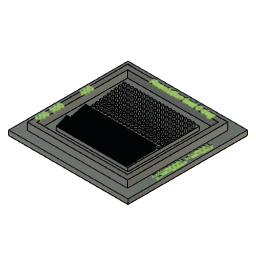
resolution_test_plate_increasing_feature_size v6 (Autodesk Fusion 360 design; units mm, degrees)
Autodesk Fusion 360 part; units mm, degrees
note: some values were not read from the file. Set by a fixed rule: which face or edge a step refers to.
(part 1 of 2)
sketch "Sketch1" plane through (0, 0, 0) normal (0, 0, 1) x (1, 0, 0)
  line L0 (0, 0) -> (-25, 0)
  line L1 (-25, 0) -> (-25, 25)
  line L2 (-25, 25) -> (0, 25)
  line L3 (0, 25) -> (0, 0)
  dimension "d1" = 25
  dimension "d2" = 25
  constraint horizontal L0
  constraint vertical L1
  constraint horizontal L2
  constraint vertical L3
  constraint coincident L0.start L3.end
  measures "d1" distance of L0.start L0.end
  measures "d2" distance of L0.start L2.end
extrude "Extrude1" add sketch "Sketch1" along normal blind 1
sketch "Sketch2" plane through (0, 0, 1) normal (0, 0, 1) x (-1, 0, 0)
  line L0 (0, -25) -> (25, -25)
  line L1 (25, -25) -> (25, 0)
  line L2 (25, 0) -> (0, 0)
  line L3 (0, 0) -> (0, -25)
  line L4 (22.9884, -22.8968) -> (1.9884, -22.8968)
  line L5 (1.9884, -22.8968) -> (1.9884, -1.8968)
  line L6 (1.9884, -1.8968) -> (22.9884, -1.8968)
  line L7 (22.9884, -1.8968) -> (22.9884, -22.8968)
  dimension "d5" = 21
  dimension "d6" = 21
  constraint horizontal L4
  constraint vertical L5
  constraint horizontal L6
  constraint vertical L7
  measures "d5" distance of L4.start L4.end
  measures "d6" distance of L4.start L6.end
extrude "Extrude2" add sketch "Sketch2" along normal blind 1.5 contours L4 L5 L6 L7
shell "Shell1" thickness 1 removed faces 1 at (-15.9884, 15.8968, 2.5)
sketch "Sketch3" plane through (0, 0, 1) normal (0, 0, 1) x (-1, 0, 0)
  line L0 (21.9884, -2.8968) -> (2.9884, -2.8968)
  line L1 (2.9884, -2.8968) -> (2.9884, -21.8968)
  line L2 (2.9884, -21.8968) -> (21.9884, -21.8968)
  line L3 (21.9884, -21.8968) -> (21.9884, -2.8968)
  line L4 (19.953, -19.9105) -> (4.953, -19.9105)
  line L5 (4.953, -19.9105) -> (4.953, -4.9105)
  line L6 (4.953, -4.9105) -> (19.953, -4.9105)
  line L7 (19.953, -4.9105) -> (19.953, -19.9105)
  dimension "d10" = 15
  dimension "d11" = 15
  constraint horizontal L4
  constraint vertical L5
  constraint horizontal L6
  constraint vertical L7
  measures "d10" distance of L4.start L4.end
  measures "d11" distance of L4.start L6.end
extrude "Extrude3" add sketch "Sketch3" along normal blind 0.75 contours L4 L5 L6 L7
sketch "Sketch6" plane through (0, 0, 1.75) normal (0, 0, 1) x (-1, 0, 0)
  line L0 (19.953, -4.9105) -> (4.953, -4.9105)
  line L1 (4.953, -4.9105) -> (4.953, -19.9105)
  line L2 (4.953, -19.9105) -> (19.953, -19.9105)
  line L3 (19.953, -19.9105) -> (19.953, -4.9105)
  line L4 (19.8995, -4.9499) -> (19.7995, -4.9499)
  line L5 (19.7995, -4.9499) -> (19.7995, -5.0499)
  line L6 (19.7995, -5.0499) -> (19.8995, -5.0499)
  line L7 (19.8995, -5.0499) -> (19.8995, -4.9499)
  dimension "d88" = 0.1
  dimension "d89" = 0.1
  constraint horizontal L4
  constraint vertical L5
  constraint horizontal L6
  constraint vertical L7
  measures "d88" distance of L4.start L4.end
  measures "d89" distance of L4.start L6.end
extrude "Extrude10" add sketch "Sketch6" along normal blind 0.1 contours L4 L5 L6 L7
pattern_linear "R-Pattern10" count 10 spacing 0.2222 along (0, 1, 0) of 5 faces at (-19.8662, 4.9499, 1.7833) (-19.8328, 5.0165, 1.85) (-19.7995, 4.9832, 1.7833) (-19.8328, 5.0499, 1.7833) (-19.8995, 5.0165, 1.7833)
extrude "Extrude11" add 1 faces at (-19.8328, 5.2387, 1.85) along direction (0, 0, 1) blind 0.1
extrude "Extrude12" add 1 faces at (-19.8328, 5.461, 1.85) along direction (0, 0, 1) blind 0.2
extrude "Extrude13" add 1 faces at (-19.8328, 5.6832, 1.85) along direction (0, 0, 1) blind 0.3
extrude "Extrude14" add 1 faces at (-19.8328, 5.9054, 1.85) along direction (0, 0, 1) blind 0.4
extrude "Extrude15" add 1 faces at (-19.8328, 6.1276, 1.85) along direction (0, 0, 1) blind 0.5
extrude "Extrude16" add 1 faces at (-19.8328, 6.3499, 1.85) along direction (0, 0, 1) blind 0.6
extrude "Extrude17" add 1 faces at (-19.8328, 6.5721, 1.85) along direction (0, 0, 1) blind 0.7
extrude "Extrude18" add 1 faces at (-19.8328, 6.7943, 1.85) along direction (0, 0, 1) blind 0.8
extrude "Extrude19" add 1 faces at (-19.8328, 7.0165, 1.85) along direction (0, 0, 1) blind 0.9
sketch "Sketch7" plane through (0, 0, 1.75) normal (0, 0, 1) x (-1, 0, 0)
  line L0 (19.8995, -7.0499) -> (19.7995, -7.0499)
  line L1 (19.7995, -7.0499) -> (19.7995, -6.9499)
  line L2 (19.7995, -6.9499) -> (19.8995, -6.9499)
  line L3 (19.8995, -6.9499) -> (19.8995, -7.0499)
  line L4 (19.8995, -6.8276) -> (19.7995, -6.8276)
  line L5 (19.7995, -6.8276) -> (19.7995, -6.7276)
  line L6 (19.7995, -6.7276) -> (19.8995, -6.7276)
  line L7 (19.8995, -6.7276) -> (19.8995, -6.8276)
  line L8 (19.8995, -6.6054) -> (19.7995, -6.6054)
  line L9 (19.7995, -6.6054) -> (19.7995, -6.5054)
  line L10 (19.7995, -6.5054) -> (19.8995, -6.5054)
  line L11 (19.8995, -6.5054) -> (19.8995, -6.6054)
  line L12 (19.8995, -6.3832) -> (19.7995, -6.3832)
  line L13 (19.7995, -6.3832) -> (19.7995, -6.2832)
  line L14 (19.7995, -6.2832) -> (19.8995, -6.2832)
  line L15 (19.8995, -6.2832) -> (19.8995, -6.3832)
  line L16 (19.8995, -6.161) -> (19.7995, -6.161)
  line L17 (19.7995, -6.161) -> (19.7995, -6.061)
  line L18 (19.7995, -6.061) -> (19.8995, -6.061)
  line L19 (19.8995, -6.061) -> (19.8995, -6.161)
  line L20 (19.8995, -5.9387) -> (19.7995, -5.9387)
  line L21 (19.7995, -5.9387) -> (19.7995, -5.8387)
  line L22 (19.7995, -5.8387) -> (19.8995, -5.8387)
  line L23 (19.8995, -5.8387) -> (19.8995, -5.9387)
  line L24 (19.8995, -5.7165) -> (19.7995, -5.7165)
  line L25 (19.7995, -5.7165) -> (19.7995, -5.6165)
  line L26 (19.7995, -5.6165) -> (19.8995, -5.6165)
  line L27 (19.8995, -5.6165) -> (19.8995, -5.7165)
  line L28 (19.8995, -5.4943) -> (19.7995, -5.4943)
  line L29 (19.7995, -5.4943) -> (19.7995, -5.3943)
  line L30 (19.7995, -5.3943) -> (19.8995, -5.3943)
  line L31 (19.8995, -5.3943) -> (19.8995, -5.4943)
  line L32 (19.8995, -5.2721) -> (19.7995, -5.2721)
  line L33 (19.7995, -5.2721) -> (19.7995, -5.1721)
  line L34 (19.7995, -5.1721) -> (19.8995, -5.1721)
  line L35 (19.8995, -5.1721) -> (19.8995, -5.2721)
  line L36 (19.8995, -5.0499) -> (19.7995, -5.0499)
  line L37 (19.7995, -5.0499) -> (19.7995, -4.9499)
  line L38 (19.7995, -4.9499) -> (19.8995, -4.9499)
  line L39 (19.8995, -4.9499) -> (19.8995, -5.0499)
  line L40 (19.953, -4.9105) -> (4.953, -4.9105)
  line L41 (4.953, -4.9105) -> (4.953, -19.9105)
  line L42 (4.953, -19.9105) -> (19.953, -19.9105)
  line L43 (19.953, -19.9105) -> (19.953, -4.9105)
  line L44 (19.8984, -7.2019) -> (19.6984, -7.2019)
  line L45 (19.6984, -7.2019) -> (19.6984, -7.4019)
  line L46 (19.6984, -7.4019) -> (19.8984, -7.4019)
  line L47 (19.8984, -7.4019) -> (19.8984, -7.2019)
  dimension "d122" = 0.2
  dimension "d123" = 0.2
  constraint horizontal L44
  constraint vertical L45
  constraint horizontal L46
  constraint vertical L47
  measures "d122" distance of L44.start L44.end
  measures "d123" distance of L44.start L46.end
extrude "Extrude20" add sketch "Sketch7" along normal blind 0.1 contours L44 L45 L46 L47
pattern_linear "R-Pattern12" count 10 spacing 0.4 along (0, 1, 0) of 5 faces at (-19.8317, 7.2019, 1.7833) (-19.7651, 7.2685, 1.85) (-19.6984, 7.2685, 1.7833) (-19.7651, 7.4019, 1.7833) (-19.8984, 7.3352, 1.7833)
sketch "Sketch8" plane through (0, 0, 1.75) normal (0, 0, 1) x (-1, 0, 0)
  line L0 (19.8984, -11.0019) -> (19.6984, -11.0019)
  line L1 (19.6984, -11.0019) -> (19.6984, -10.8019)
  line L2 (19.6984, -10.8019) -> (19.8984, -10.8019)
  line L3 (19.8984, -10.8019) -> (19.8984, -11.0019)
  line L4 (19.8984, -10.6019) -> (19.6984, -10.6019)
  line L5 (19.6984, -10.6019) -> (19.6984, -10.4019)
  line L6 (19.6984, -10.4019) -> (19.8984, -10.4019)
  line L7 (19.8984, -10.4019) -> (19.8984, -10.6019)
  line L8 (19.8984, -10.2019) -> (19.6984, -10.2019)
  line L9 (19.6984, -10.2019) -> (19.6984, -10.0019)
  line L10 (19.6984, -10.0019) -> (19.8984, -10.0019)
  line L11 (19.8984, -10.0019) -> (19.8984, -10.2019)
  line L12 (19.8984, -9.8019) -> (19.6984, -9.8019)
  line L13 (19.6984, -9.8019) -> (19.6984, -9.6019)
  line L14 (19.6984, -9.6019) -> (19.8984, -9.6019)
  line L15 (19.8984, -9.6019) -> (19.8984, -9.8019)
  line L16 (19.8984, -9.4019) -> (19.6984, -9.4019)
  line L17 (19.6984, -9.4019) -> (19.6984, -9.2019)
  line L18 (19.6984, -9.2019) -> (19.8984, -9.2019)
  line L19 (19.8984, -9.2019) -> (19.8984, -9.4019)
  line L20 (19.8984, -9.0019) -> (19.6984, -9.0019)
  line L21 (19.6984, -9.0019) -> (19.6984, -8.8019)
  line L22 (19.6984, -8.8019) -> (19.8984, -8.8019)
  line L23 (19.8984, -8.8019) -> (19.8984, -9.0019)
  line L24 (19.8984, -8.6019) -> (19.6984, -8.6019)
  line L25 (19.6984, -8.6019) -> (19.6984, -8.4019)
  line L26 (19.6984, -8.4019) -> (19.8984, -8.4019)
  line L27 (19.8984, -8.4019) -> (19.8984, -8.6019)
  line L28 (19.8984, -8.2019) -> (19.6984, -8.2019)
  line L29 (19.6984, -8.2019) -> (19.6984, -8.0019)
  line L30 (19.6984, -8.0019) -> (19.8984, -8.0019)
  line L31 (19.8984, -8.0019) -> (19.8984, -8.2019)
  line L32 (19.8984, -7.8019) -> (19.6984, -7.8019)
  line L33 (19.6984, -7.8019) -> (19.6984, -7.6019)
  line L34 (19.6984, -7.6019) -> (19.8984, -7.6019)
  line L35 (19.8984, -7.6019) -> (19.8984, -7.8019)
  line L36 (19.8984, -7.4019) -> (19.6984, -7.4019)
  line L37 (19.6984, -7.4019) -> (19.6984, -7.2019)
  line L38 (19.6984, -7.2019) -> (19.8984, -7.2019)
  line L39 (19.8984, -7.2019) -> (19.8984, -7.4019)
  line L40 (19.8995, -7.0499) -> (19.7995, -7.0499)
  line L41 (19.7995, -7.0499) -> (19.7995, -6.9499)
  line L42 (19.7995, -6.9499) -> (19.8995, -6.9499)
  line L43 (19.8995, -6.9499) -> (19.8995, -7.0499)
  line L44 (19.8995, -6.8276) -> (19.7995, -6.8276)
  line L45 (19.7995, -6.8276) -> (19.7995, -6.7276)
  line L46 (19.7995, -6.7276) -> (19.8995, -6.7276)
  line L47 (19.8995, -6.7276) -> (19.8995, -6.8276)
  line L48 (19.8995, -6.6054) -> (19.7995, -6.6054)
  line L49 (19.7995, -6.6054) -> (19.7995, -6.5054)
  line L50 (19.7995, -6.5054) -> (19.8995, -6.5054)
  line L51 (19.8995, -6.5054) -> (19.8995, -6.6054)
  line L52 (19.8995, -6.3832) -> (19.7995, -6.3832)
  line L53 (19.7995, -6.3832) -> (19.7995, -6.2832)
  line L54 (19.7995, -6.2832) -> (19.8995, -6.2832)
  line L55 (19.8995, -6.2832) -> (19.8995, -6.3832)
  line L56 (19.8995, -6.161) -> (19.7995, -6.161)
  line L57 (19.7995, -6.161) -> (19.7995, -6.061)
  line L58 (19.7995, -6.061) -> (19.8995, -6.061)
  line L59 (19.8995, -6.061) -> (19.8995, -6.161)
  line L60 (19.8995, -5.9387) -> (19.7995, -5.9387)
  line L61 (19.7995, -5.9387) -> (19.7995, -5.8387)
  line L62 (19.7995, -5.8387) -> (19.8995, -5.8387)
  line L63 (19.8995, -5.8387) -> (19.8995, -5.9387)
  line L64 (19.8995, -5.7165) -> (19.7995, -5.7165)
  line L65 (19.7995, -5.7165) -> (19.7995, -5.6165)
  line L66 (19.7995, -5.6165) -> (19.8995, -5.6165)
  line L67 (19.8995, -5.6165) -> (19.8995, -5.7165)
  line L68 (19.8995, -5.4943) -> (19.7995, -5.4943)
  line L69 (19.7995, -5.4943) -> (19.7995, -5.3943)
  line L70 (19.7995, -5.3943) -> (19.8995, -5.3943)
  line L71 (19.8995, -5.3943) -> (19.8995, -5.4943)
  line L72 (19.8995, -5.2721) -> (19.7995, -5.2721)
  line L73 (19.7995, -5.2721) -> (19.7995, -5.1721)
  line L74 (19.7995, -5.1721) -> (19.8995, -5.1721)
  line L75 (19.8995, -5.1721) -> (19.8995, -5.2721)
  line L76 (19.8995, -5.0499) -> (19.7995, -5.0499)
  line L77 (19.7995, -5.0499) -> (19.7995, -4.9499)
  line L78 (19.7995, -4.9499) -> (19.8995, -4.9499)
  line L79 (19.8995, -4.9499) -> (19.8995, -5.0499)
  line L80 (19.953, -4.9105) -> (4.953, -4.9105)
  line L81 (4.953, -4.9105) -> (4.953, -19.9105)
  line L82 (4.953, -19.9105) -> (19.953, -19.9105)
  line L83 (19.953, -19.9105) -> (19.953, -4.9105)
  line L84 (19.899, -11.503) -> (19.499, -11.503)
  line L85 (19.499, -11.503) -> (19.499, -11.903)
  line L86 (19.499, -11.903) -> (19.899, -11.903)
  line L87 (19.899, -11.903) -> (19.899, -11.503)
  dimension "d130" = 0.4
  dimension "d131" = 0.4
  constraint horizontal L84
  constraint vertical L85
  constraint horizontal L86
  constraint vertical L87
  measures "d130" distance of L84.start L84.end
  measures "d131" distance of L84.start L86.end
extrude "Extrude21" add sketch "Sketch8" along normal blind 0.1 contours L84 L85 L86 L87
pattern_linear "R-Pattern13" count 10 spacing 0.8 along (0, 1, 0) of 5 faces at (-19.6323, 11.6364, 1.85) (-19.7657, 11.503, 1.7833) (-19.499, 11.6364, 1.7833) (-19.6323, 11.903, 1.7833) (-19.899, 11.7697, 1.7833)
extrude "Extrude22" add 1 faces at (-19.7651, 7.6685, 1.85) along direction (0, 0, 1) blind 0.1
extrude "Extrude23" add 1 faces at (-19.7651, 8.0685, 1.85) along direction (0, 0, 1) blind 0.2
extrude "Extrude24" add 1 faces at (-19.7651, 8.4685, 1.85) along direction (0, 0, 1) blind 0.3
extrude "Extrude25" add 1 faces at (-19.7651, 8.8685, 1.85) along direction (0, 0, 1) blind 0.4
extrude "Extrude26" add 1 faces at (-19.7651, 9.2685, 1.85) along direction (0, 0, 1) blind 0.5
extrude "Extrude27" add 1 faces at (-19.7651, 9.6685, 1.85) along direction (0, 0, 1) blind 0.6
extrude "Extrude28" add 1 faces at (-19.7651, 10.0685, 1.85) along direction (0, 0, 1) blind 0.7
extrude "Extrude29" add 1 faces at (-19.7651, 10.4685, 1.85) along direction (0, 0, 1) blind 0.8
extrude "Extrude30" add 1 faces at (-19.7651, 10.8685, 1.85) along direction (0, 0, 1) blind 0.9
extrude "Extrude31" add 1 faces at (-19.6323, 12.4364, 1.85) along direction (0, 0, 1) blind 0.1
extrude "Extrude32" add 1 faces at (-19.6323, 13.2364, 1.85) along direction (0, 0, 1) blind 0.2
extrude "Extrude33" add 1 faces at (-19.6323, 14.0364, 1.85) along direction (0, 0, 1) blind 0.3
extrude "Extrude34" add 1 faces at (-19.6323, 14.8364, 1.85) along direction (0, 0, 1) blind 0.4
extrude "Extrude35" add 1 faces at (-19.6323, 15.6364, 1.85) along direction (0, 0, 1) blind 0.5
extrude "Extrude36" add 1 faces at (-19.6323, 16.4364, 1.85) along direction (0, 0, 1) blind 0.6
extrude "Extrude37" add 1 faces at (-19.6323, 17.2364, 1.85) along direction (0, 0, 1) blind 0.7
extrude "Extrude38" add 1 faces at (-19.6323, 18.0364, 1.85) along direction (0, 0, 1) blind 0.8
extrude "Extrude39" add 1 faces at (-19.6323, 18.8364, 1.85) along direction (0, 0, 1) blind 0.9
pattern_linear "R-Pattern14" count 19 spacing 0.8 along (1, 0, 0) of 50 faces at (-19.6323, 18.703, 2.4167) (-19.499, 18.9697, 2.4167) (-19.6323, 18.8364, 2.75) (-19.499, 18.0364, 2.35) (-19.6323, 17.903, 2.35) (-19.6323, 18.0364, 2.65) (-19.6323, 17.2364, 2.55) (-19.6323, 17.103, 2.2833) (-19.499, 17.3697, 2.2833) (-19.499, 16.4364, 2.2167) (-19.6323, 16.303, 2.2167) (-19.6323, 16.4364, 2.45) (-19.6323, 15.6364, 2.35) (-19.499, 15.7697, 2.15) (-19.6323, 15.503, 2.15) (-19.499, 14.9697, 2.0833) (-19.6323, 14.703, 2.0833) (-19.6323, 14.8364, 2.25) (-19.6323, 14.0364, 2.15) (-19.499, 14.1697, 2.0167) (-19.6323, 13.903, 2.0167) (-19.499, 13.3697, 1.95) (-19.6323, 13.103, 1.95) (-19.6323, 13.2364, 2.05) (-19.6323, 12.4364, 1.95) (-19.499, 12.5697, 1.8833) (-19.6323, 12.303, 1.8833) (-19.6323, 11.6364, 1.85) (-19.7657, 11.503, 1.7833) (-19.499, 11.6364, 1.7833) (-19.899, 11.7697, 1.7833) (-19.6323, 11.903, 1.7833) (-19.899, 12.5697, 1.8167) (-19.6323, 12.703, 1.8167) (-19.899, 13.3697, 1.85) (-19.6323, 13.503, 1.85) (-19.899, 14.1697, 1.8833) (-19.6323, 14.303, 1.8833) (-19.899, 14.9697, 1.9167) (-19.6323, 15.103, 1.9167) (-19.899, 15.7697, 1.95) (-19.6323, 15.903, 1.95) (-19.899, 16.5697, 2.2167) (-19.6323, 16.703, 1.9833) (-19.899, 17.3697, 2.0167) (-19.6323, 17.503, 2.0167) (-19.899, 18.1697, 2.35) (-19.6323, 18.303, 2.05) (-19.899, 18.9697, 2.0833) (-19.6323, 19.103, 2.0833)
pattern_linear "R-Pattern15" count 37 spacing 0.4 along (1, 0, 0) of 50 faces at (-19.6984, 10.9352, 2.4167) (-19.7651, 10.8685, 2.75) (-19.7651, 10.8019, 2.4167) (-19.6984, 10.5352, 2.35) (-19.7651, 10.4685, 2.65) (-19.7651, 10.4019, 2.35) (-19.6984, 10.1352, 2.2833) (-19.7651, 10.0685, 2.55) (-19.7651, 10.0019, 2.2833) (-19.6984, 9.7352, 2.2167) (-19.7651, 9.6685, 2.45) (-19.7651, 9.6019, 2.2167) (-19.6984, 9.3352, 2.15) (-19.7651, 9.2019, 2.15) (-19.7651, 9.2685, 2.35) (-19.6984, 8.9352, 2.0833) (-19.7651, 8.8019, 2.0833) (-19.7651, 8.8685, 2.25) (-19.6984, 8.5352, 2.0167) (-19.7651, 8.4019, 2.0167) (-19.7651, 8.4685, 2.15) (-19.6984, 8.0685, 1.95) (-19.7651, 8.0019, 1.95) (-19.7651, 8.0685, 2.05) (-19.6984, 7.7352, 1.8833) (-19.7651, 7.6019, 1.8833) (-19.7651, 7.6685, 1.95) (-19.6984, 7.2685, 1.7833) (-19.8317, 7.2019, 1.7833) (-19.7651, 7.2685, 1.85) (-19.7651, 11.0019, 2.0833) (-19.8984, 10.9352, 2.0833) (-19.7651, 10.6019, 2.05) (-19.8984, 10.5352, 2.05) (-19.7651, 10.2019, 2.0167) (-19.8984, 10.1352, 2.0167) (-19.7651, 9.8019, 1.9833) (-19.8984, 9.7352, 1.9833) (-19.7651, 9.4019, 1.95) (-19.8984, 9.3352, 1.95) (-19.7651, 9.0019, 1.9167) (-19.8984, 8.9352, 1.9167) (-19.7651, 8.6019, 1.8833) (-19.8984, 8.5352, 1.8833) (-19.7651, 8.2019, 1.85) (-19.8984, 8.1352, 1.95) (-19.7651, 7.8019, 1.8167) (-19.8984, 7.7352, 1.8167) (-19.7651, 7.4019, 1.7833) (-19.8984, 7.3352, 1.7833)
pattern_linear "R-Pattern16" count 74 spacing 0.2 along (1, 0, 0) of 50 faces at (-19.8662, 4.9499, 1.7833) (-19.7995, 4.9832, 1.7833) (-19.8328, 5.0165, 1.85) (-19.8328, 5.1721, 1.8833) (-19.8328, 5.2387, 1.95) (-19.7995, 5.2387, 1.8833) (-19.8328, 5.3943, 1.95) (-19.8328, 5.461, 2.05) (-19.7995, 5.461, 1.95) (-19.8328, 5.6165, 2.0167) (-19.8328, 5.6832, 2.15) (-19.7995, 5.6832, 2.0167) (-19.8328, 5.8387, 2.0833) (-19.8328, 5.9054, 2.25) (-19.7995, 5.9054, 2.0833) (-19.8328, 6.061, 2.15) (-19.8328, 6.1276, 2.35) (-19.7995, 6.1276, 2.15) (-19.8328, 6.2832, 2.2167) (-19.8328, 6.3499, 2.45) (-19.7995, 6.3499, 2.2167) (-19.8328, 6.5054, 2.2833) (-19.8328, 6.5721, 2.55) (-19.7995, 6.5721, 2.2833) (-19.8328, 6.7276, 2.35) (-19.8328, 6.7943, 2.65) (-19.7995, 6.7943, 2.35) (-19.8328, 6.9499, 2.4167) (-19.8328, 7.0165, 2.75) (-19.7995, 7.0165, 2.4167) (-19.8995, 5.0165, 1.7833) (-19.8328, 5.0499, 1.7833) (-19.8995, 5.2387, 1.8167) (-19.8328, 5.2721, 1.8167) (-19.8995, 5.461, 1.85) (-19.8328, 5.4943, 1.85) (-19.8328, 5.7165, 1.8833) (-19.8995, 5.6832, 1.8833) (-19.8995, 5.9054, 1.9167) (-19.8328, 5.9387, 1.9167) (-19.8995, 6.1276, 1.95) (-19.8328, 6.161, 1.95) (-19.8995, 6.3499, 1.9833) (-19.8328, 6.3832, 1.9833) (-19.8995, 6.5721, 2.0167) (-19.8328, 6.6054, 2.0167) (-19.8995, 6.7943, 2.05) (-19.8328, 6.8276, 2.05) (-19.8995, 7.0165, 2.0833) (-19.8328, 7.0499, 2.0833)
sketch "Sketch9" plane through (0, 0, 1) normal (0, 0, 1) x (-1, 0, 0)
  line L0 (22.9884, -1.8968) -> (22.9884, -22.8968)
  line L1 (22.9884, -22.8968) -> (1.9884, -22.8968)
  line L2 (1.9884, -22.8968) -> (1.9884, -1.8968)
  line L3 (1.9884, -1.8968) -> (22.9884, -1.8968)
  line L4 (0, -25) -> (25, -25)
  line L5 (25, -25) -> (25, 0)
  line L6 (25, 0) -> (0, 0)
  line L7 (0, 0) -> (0, -25)
  line L8 (24.5135, -24.4817) -> (23.4918, -24.4817)
  line L9 (23.4918, -24.4817) -> (23.4918, -23.5086)
  line L10 (23.4918, -23.5086) -> (24.5135, -23.5086)
  line L11 (24.5135, -23.5086) -> (24.5135, -24.4817)
  constraint horizontal L8
  constraint vertical L9
  constraint horizontal L10
  constraint vertical L11
extrude "Extrude40" cut sketch "Sketch9" against normal blind 0.5 contours L8 L9 L10 L11
sketch "Sketch10" plane through (0, 0, 1) normal (0, 0, 1) x (-1, 0, 0)
  line L0 (23.4918, -24.4817) -> (23.4918, -23.5086)
  line L1 (23.4918, -23.5086) -> (24.5135, -23.5086)
  line L2 (24.5135, -23.5086) -> (24.5135, -24.4817)
  line L3 (24.5135, -24.4817) -> (23.4918, -24.4817)
  line L4 (22.9884, -1.8968) -> (22.9884, -22.8968)
  line L5 (22.9884, -22.8968) -> (1.9884, -22.8968)
  line L6 (1.9884, -22.8968) -> (1.9884, -1.8968)
  line L7 (1.9884, -1.8968) -> (22.9884, -1.8968)
  line L8 (0, -25) -> (25, -25)
  line L9 (25, -25) -> (25, 0)
  line L10 (25, 0) -> (0, 0)
  line L11 (0, 0) -> (0, -25)
  line L12 (1.4942, -17.9711) -> (1.4942, -18.0939)
  line L13 (1.4942, -18.0939) -> (0.7118, -18.0939)
  spline S0 degree 2 poles (0.7118, -18.0939) (0.7541, -18.1382) (0.7964, -18.2102) knots 0 0 0 1 1 1
  spline S1 degree 2 poles (0.7964, -18.2102) (0.8387, -18.2821) (0.8598, -18.3394) knots 0 0 0 1 1 1
  line L14 (0.8598, -18.3394) -> (0.7411, -18.3394)
  spline S2 degree 2 poles (0.7411, -18.3394) (0.6927, -18.2364) (0.6238, -18.1593) knots 0 0 0 1 1 1
  spline S3 degree 2 poles (0.6238, -18.1593) (0.5549, -18.0823) (0.4901, -18.0502) knots 0 0 0 1 1 1
  line L15 (0.4901, -18.0502) -> (0.4901, -17.9711)
  line L16 (0.4901, -17.9711) -> (1.4942, -17.9711)
  spline S4 degree 2 poles (1.001, -17.6566) (0.8237, -17.6566) (0.7156, -17.6201) knots 0 0 0 1 1 1
  spline S5 degree 2 poles (0.7156, -17.6201) (0.6074, -17.5836) (0.5488, -17.5117) knots 0 0 0 1 1 1
  spline S6 degree 2 poles (0.5488, -17.5117) (0.4901, -17.4397) (0.4901, -17.3306) knots 0 0 0 1 1 1
  spline S7 degree 2 poles (0.4901, -17.3306) (0.4901, -17.2501) (0.5225, -17.1894) knots 0 0 0 1 1 1
  spline S8 degree 2 poles (0.5225, -17.1894) (0.5549, -17.1286) (0.616, -17.0891) knots 0 0 0 1 1 1
  spline S9 degree 2 poles (0.616, -17.0891) (0.677, -17.0495) (0.7647, -17.027) knots 0 0 0 1 1 1
  spline S10 degree 2 poles (0.7647, -17.027) (0.8523, -17.0045) (1.001, -17.0045) knots 0 0 0 1 1 1
  spline S11 degree 2 poles (1.001, -17.0045) (1.177, -17.0045) (1.2851, -17.0406) knots 0 0 0 1 1 1
  spline S12 degree 2 poles (1.2851, -17.0406) (1.3933, -17.0768) (1.4523, -17.1488) knots 0 0 0 1 1 1
  spline S13 degree 2 poles (1.4523, -17.1488) (1.5113, -17.2207) (1.5113, -17.3306) knots 0 0 0 1 1 1
  spline S14 degree 2 poles (1.5113, -17.3306) (1.5113, -17.4752) (1.4076, -17.5577) knots 0 0 0 1 1 1
  spline S15 degree 2 poles (1.4076, -17.5577) (1.2827, -17.6566) (1.001, -17.6566) knots 0 0 0 1 1 1
  spline S16 degree 2 poles (1.001, -17.5304) (1.2473, -17.5304) (1.3288, -17.4728) knots 0 0 0 1 1 1
  spline S17 degree 2 poles (1.3288, -17.4728) (1.4103, -17.4151) (1.4103, -17.3306) knots 0 0 0 1 1 1
  spline S18 degree 2 poles (1.4103, -17.3306) (1.4103, -17.246) (1.3284, -17.1883) knots 0 0 0 1 1 1
  spline S19 degree 2 poles (1.3284, -17.1883) (1.2466, -17.1307) (1.001, -17.1307) knots 0 0 0 1 1 1
  spline S20 degree 2 poles (1.001, -17.1307) (0.7541, -17.1307) (0.6729, -17.1883) knots 0 0 0 1 1 1
  spline S21 degree 2 poles (0.6729, -17.1883) (0.5917, -17.246) (0.5917, -17.3319) knots 0 0 0 1 1 1
  spline S22 degree 2 poles (0.5917, -17.3319) (0.5917, -17.4165) (0.6634, -17.467) knots 0 0 0 1 1 1
  spline S23 degree 2 poles (0.6634, -17.467) (0.7548, -17.5304) (1.001, -17.5304) knots 0 0 0 1 1 1
  spline S24 degree 2 poles (1.001, -16.8797) (0.8237, -16.8797) (0.7156, -16.8432) knots 0 0 0 1 1 1
  spline S25 degree 2 poles (0.7156, -16.8432) (0.6074, -16.8067) (0.5488, -16.7347) knots 0 0 0 1 1 1
  spline S26 degree 2 poles (0.5488, -16.7347) (0.4901, -16.6628) (0.4901, -16.5536) knots 0 0 0 1 1 1
  spline S27 degree 2 poles (0.4901, -16.5536) (0.4901, -16.4731) (0.5225, -16.4124) knots 0 0 0 1 1 1
  spline S28 degree 2 poles (0.5225, -16.4124) (0.5549, -16.3517) (0.616, -16.3121) knots 0 0 0 1 1 1
  spline S29 degree 2 poles (0.616, -16.3121) (0.677, -16.2726) (0.7647, -16.2501) knots 0 0 0 1 1 1
  spline S30 degree 2 poles (0.7647, -16.2501) (0.8523, -16.2276) (1.001, -16.2276) knots 0 0 0 1 1 1
  spline S31 degree 2 poles (1.001, -16.2276) (1.177, -16.2276) (1.2851, -16.2637) knots 0 0 0 1 1 1
  spline S32 degree 2 poles (1.2851, -16.2637) (1.3933, -16.2999) (1.4523, -16.3718) knots 0 0 0 1 1 1
  spline S33 degree 2 poles (1.4523, -16.3718) (1.5113, -16.4438) (1.5113, -16.5536) knots 0 0 0 1 1 1
  spline S34 degree 2 poles (1.5113, -16.5536) (1.5113, -16.6982) (1.4076, -16.7808) knots 0 0 0 1 1 1
  spline S35 degree 2 poles (1.4076, -16.7808) (1.2827, -16.8797) (1.001, -16.8797) knots 0 0 0 1 1 1
  spline S36 degree 2 poles (1.001, -16.7535) (1.2473, -16.7535) (1.3288, -16.6958) knots 0 0 0 1 1 1
  spline S37 degree 2 poles (1.3288, -16.6958) (1.4103, -16.6382) (1.4103, -16.5536) knots 0 0 0 1 1 1
  spline S38 degree 2 poles (1.4103, -16.5536) (1.4103, -16.469) (1.3284, -16.4114) knots 0 0 0 1 1 1
  spline S39 degree 2 poles (1.3284, -16.4114) (1.2466, -16.3537) (1.001, -16.3537) knots 0 0 0 1 1 1
  spline S40 degree 2 poles (1.001, -16.3537) (0.7541, -16.3537) (0.6729, -16.4114) knots 0 0 0 1 1 1
  spline S41 degree 2 poles (0.6729, -16.4114) (0.5917, -16.469) (0.5917, -16.555) knots 0 0 0 1 1 1
  spline S42 degree 2 poles (0.5917, -16.555) (0.5917, -16.6396) (0.6634, -16.69) knots 0 0 0 1 1 1
  spline S43 degree 2 poles (0.6634, -16.69) (0.7548, -16.7535) (1.001, -16.7535) knots 0 0 0 1 1 1
  line L17 (1.4942, -15.5939) -> (1.3878, -15.5939)
  spline S44 degree 2 poles (1.3878, -15.5939) (1.5106, -15.6784) (1.5106, -15.8237) knots 0 0 0 1 1 1
  spline S45 degree 2 poles (1.5106, -15.8237) (1.5106, -15.8879) (1.486, -15.9434) knots 0 0 0 1 1 1
  spline S46 degree 2 poles (1.486, -15.9434) (1.4615, -15.999) (1.4243, -16.026) knots 0 0 0 1 1 1
  spline S47 degree 2 poles (1.4243, -16.026) (1.3871, -16.0529) (1.3332, -16.0638) knots 0 0 0 1 1 1
  spline S48 degree 2 poles (1.3332, -16.0638) (1.2971, -16.0713) (1.2186, -16.0713) knots 0 0 0 1 1 1
  line L18 (1.2186, -16.0713) -> (0.7698, -16.0713)
  line L19 (0.7698, -16.0713) -> (0.7698, -15.9486)
  line L20 (0.7698, -15.9486) -> (1.1716, -15.9486)
  spline S49 degree 2 poles (1.1716, -15.9486) (1.2677, -15.9486) (1.3012, -15.9411) knots 0 0 0 1 1 1
  spline S50 degree 2 poles (1.3012, -15.9411) (1.3496, -15.9295) (1.3772, -15.8919) knots 0 0 0 1 1 1
  spline S51 degree 2 poles (1.3772, -15.8919) (1.4048, -15.8544) (1.4048, -15.7992) knots 0 0 0 1 1 1
  spline S52 degree 2 poles (1.4048, -15.7992) (1.4048, -15.7439) (1.3765, -15.6955) knots 0 0 0 1 1 1
  spline S53 degree 2 poles (1.3765, -15.6955) (1.3482, -15.6471) (1.2995, -15.6269) knots 0 0 0 1 1 1
  spline S54 degree 2 poles (1.2995, -15.6269) (1.2507, -15.6068) (1.1579, -15.6068) knots 0 0 0 1 1 1
  line L21 (1.1579, -15.6068) -> (0.7698, -15.6068)
  line L22 (0.7698, -15.6068) -> (0.7698, -15.484)
  line L23 (0.7698, -15.484) -> (1.4942, -15.484)
  line L24 (1.4942, -15.484) -> (1.4942, -15.5939)
  line L25 (1.4942, -15.2917) -> (0.7698, -15.2917)
  line L26 (0.7698, -15.2917) -> (0.7698, -15.1818)
  line L27 (0.7698, -15.1818) -> (0.8714, -15.1818)
  spline S55 degree 2 poles (0.8714, -15.1818) (0.8182, -15.1477) (0.7858, -15.0911) knots 0 0 0 1 1 1
  spline S56 degree 2 poles (0.7858, -15.0911) (0.7534, -15.0345) (0.7534, -14.9622) knots 0 0 0 1 1 1
  spline S57 degree 2 poles (0.7534, -14.9622) (0.7534, -14.8817) (0.7868, -14.8302) knots 0 0 0 1 1 1
  spline S58 degree 2 poles (0.7868, -14.8302) (0.8203, -14.7787) (0.8803, -14.7576) knots 0 0 0 1 1 1
  spline S59 degree 2 poles (0.8803, -14.7576) (0.7534, -14.6716) (0.7534, -14.5338) knots 0 0 0 1 1 1
  spline S60 degree 2 poles (0.7534, -14.5338) (0.7534, -14.4261) (0.8131, -14.3681) knots 0 0 0 1 1 1
  spline S61 degree 2 poles (0.8131, -14.3681) (0.8728, -14.3101) (0.9969, -14.3101) knots 0 0 0 1 1 1
  line L28 (0.9969, -14.3101) -> (1.4942, -14.3101)
  line L29 (1.4942, -14.3101) -> (1.4942, -14.4322)
  line L30 (1.4942, -14.4322) -> (1.0379, -14.4322)
  spline S62 degree 2 poles (1.0379, -14.4322) (0.9642, -14.4322) (0.9318, -14.4441) knots 0 0 0 1 1 1
  spline S63 degree 2 poles (0.9318, -14.4441) (0.8994, -14.4561) (0.8796, -14.4874) knots 0 0 0 1 1 1
  spline S64 degree 2 poles (0.8796, -14.4874) (0.8598, -14.5188) (0.8598, -14.5611) knots 0 0 0 1 1 1
  spline S65 degree 2 poles (0.8598, -14.5611) (0.8598, -14.6375) (0.9106, -14.688) knots 0 0 0 1 1 1
  spline S66 degree 2 poles (0.9106, -14.688) (0.9615, -14.7385) (1.0733, -14.7385) knots 0 0 0 1 1 1
  line L31 (1.0733, -14.7385) -> (1.4942, -14.7385)
  line L32 (1.4942, -14.7385) -> (1.4942, -14.8612)
  line L33 (1.4942, -14.8612) -> (1.0235, -14.8612)
  spline S67 degree 2 poles (1.0235, -14.8612) (0.9417, -14.8612) (0.9008, -14.8913) knots 0 0 0 1 1 1
  spline S68 degree 2 poles (0.9008, -14.8913) (0.8598, -14.9213) (0.8598, -14.9895) knots 0 0 0 1 1 1
  spline S69 degree 2 poles (0.8598, -14.9895) (0.8598, -15.0413) (0.8871, -15.0853) knots 0 0 0 1 1 1
  spline S70 degree 2 poles (0.8871, -15.0853) (0.9144, -15.1293) (0.9669, -15.1491) knots 0 0 0 1 1 1
  spline S71 degree 2 poles (0.9669, -15.1491) (1.0194, -15.1689) (1.1184, -15.1689) knots 0 0 0 1 1 1
  line L34 (1.1184, -15.1689) -> (1.4942, -15.1689)
  line L35 (1.4942, -15.1689) -> (1.4942, -15.2917)
  line L36 (1.1941, -13.7876) -> (1.0706, -13.7876)
  line L37 (1.0706, -13.7876) -> (1.0706, -13.4104)
  line L38 (1.0706, -13.4104) -> (1.1941, -13.4104)
  line L39 (1.1941, -13.4104) -> (1.1941, -13.7876)
  line L40 (1.4942, -12.4581) -> (1.4942, -12.5809)
  line L41 (1.4942, -12.5809) -> (0.7118, -12.5809)
  spline S72 degree 2 poles (0.7118, -12.5809) (0.7541, -12.6252) (0.7964, -12.6972) knots 0 0 0 1 1 1
  spline S73 degree 2 poles (0.7964, -12.6972) (0.8387, -12.7692) (0.8598, -12.8265) knots 0 0 0 1 1 1
  line L42 (0.8598, -12.8265) -> (0.7411, -12.8265)
  spline S74 degree 2 poles (0.7411, -12.8265) (0.6927, -12.7235) (0.6238, -12.6464) knots 0 0 0 1 1 1
  spline S75 degree 2 poles (0.6238, -12.6464) (0.5549, -12.5693) (0.4901, -12.5372) knots 0 0 0 1 1 1
  line L43 (0.4901, -12.5372) -> (0.4901, -12.4581)
  line L44 (0.4901, -12.4581) -> (1.4942, -12.4581)
  spline S76 degree 2 poles (1.001, -12.1437) (0.8237, -12.1437) (0.7156, -12.1072) knots 0 0 0 1 1 1
  spline S77 degree 2 poles (0.7156, -12.1072) (0.6074, -12.0707) (0.5488, -11.9987) knots 0 0 0 1 1 1
  spline S78 degree 2 poles (0.5488, -11.9987) (0.4901, -11.9267) (0.4901, -11.8176) knots 0 0 0 1 1 1
  spline S79 degree 2 poles (0.4901, -11.8176) (0.4901, -11.7371) (0.5225, -11.6764) knots 0 0 0 1 1 1
  spline S80 degree 2 poles (0.5225, -11.6764) (0.5549, -11.6157) (0.616, -11.5761) knots 0 0 0 1 1 1
  spline S81 degree 2 poles (0.616, -11.5761) (0.677, -11.5366) (0.7647, -11.514) knots 0 0 0 1 1 1
  spline S82 degree 2 poles (0.7647, -11.514) (0.8523, -11.4915) (1.001, -11.4915) knots 0 0 0 1 1 1
  spline S83 degree 2 poles (1.001, -11.4915) (1.177, -11.4915) (1.2851, -11.5277) knots 0 0 0 1 1 1
  spline S84 degree 2 poles (1.2851, -11.5277) (1.3933, -11.5638) (1.4523, -11.6358) knots 0 0 0 1 1 1
  spline S85 degree 2 poles (1.4523, -11.6358) (1.5113, -11.7078) (1.5113, -11.8176) knots 0 0 0 1 1 1
  spline S86 degree 2 poles (1.5113, -11.8176) (1.5113, -11.9622) (1.4076, -12.0447) knots 0 0 0 1 1 1
  spline S87 degree 2 poles (1.4076, -12.0447) (1.2827, -12.1437) (1.001, -12.1437) knots 0 0 0 1 1 1
  spline S88 degree 2 poles (1.001, -12.0175) (1.2473, -12.0175) (1.3288, -11.9598) knots 0 0 0 1 1 1
  spline S89 degree 2 poles (1.3288, -11.9598) (1.4103, -11.9022) (1.4103, -11.8176) knots 0 0 0 1 1 1
  spline S90 degree 2 poles (1.4103, -11.8176) (1.4103, -11.733) (1.3284, -11.6754) knots 0 0 0 1 1 1
  spline S91 degree 2 poles (1.3284, -11.6754) (1.2466, -11.6177) (1.001, -11.6177) knots 0 0 0 1 1 1
  spline S92 degree 2 poles (1.001, -11.6177) (0.7541, -11.6177) (0.6729, -11.6754) knots 0 0 0 1 1 1
  spline S93 degree 2 poles (0.6729, -11.6754) (0.5917, -11.733) (0.5917, -11.819) knots 0 0 0 1 1 1
  spline S94 degree 2 poles (0.5917, -11.819) (0.5917, -11.9035) (0.6634, -11.954) knots 0 0 0 1 1 1
  spline S95 degree 2 poles (0.6634, -11.954) (0.7548, -12.0175) (1.001, -12.0175) knots 0 0 0 1 1 1
  spline S96 degree 2 poles (1.001, -11.3667) (0.8237, -11.3667) (0.7156, -11.3302) knots 0 0 0 1 1 1
  spline S97 degree 2 poles (0.7156, -11.3302) (0.6074, -11.2937) (0.5488, -11.2218) knots 0 0 0 1 1 1
  spline S98 degree 2 poles (0.5488, -11.2218) (0.4901, -11.1498) (0.4901, -11.0406) knots 0 0 0 1 1 1
  spline S99 degree 2 poles (0.4901, -11.0406) (0.4901, -10.9602) (0.5225, -10.8994) knots 0 0 0 1 1 1
  spline S100 degree 2 poles (0.5225, -10.8994) (0.5549, -10.8387) (0.616, -10.7992) knots 0 0 0 1 1 1
  spline S101 degree 2 poles (0.616, -10.7992) (0.677, -10.7596) (0.7647, -10.7371) knots 0 0 0 1 1 1
  spline S102 degree 2 poles (0.7647, -10.7371) (0.8523, -10.7146) (1.001, -10.7146) knots 0 0 0 1 1 1
  spline S103 degree 2 poles (1.001, -10.7146) (1.177, -10.7146) (1.2851, -10.7507) knots 0 0 0 1 1 1
  spline S104 degree 2 poles (1.2851, -10.7507) (1.3933, -10.7869) (1.4523, -10.8589) knots 0 0 0 1 1 1
  spline S105 degree 2 poles (1.4523, -10.8589) (1.5113, -10.9308) (1.5113, -11.0406) knots 0 0 0 1 1 1
  spline S106 degree 2 poles (1.5113, -11.0406) (1.5113, -11.1853) (1.4076, -11.2678) knots 0 0 0 1 1 1
  spline S107 degree 2 poles (1.4076, -11.2678) (1.2827, -11.3667) (1.001, -11.3667) knots 0 0 0 1 1 1
  spline S108 degree 2 poles (1.001, -11.2405) (1.2473, -11.2405) (1.3288, -11.1829) knots 0 0 0 1 1 1
  spline S109 degree 2 poles (1.3288, -11.1829) (1.4103, -11.1252) (1.4103, -11.0406) knots 0 0 0 1 1 1
  spline S110 degree 2 poles (1.4103, -11.0406) (1.4103, -10.9561) (1.3284, -10.8984) knots 0 0 0 1 1 1
  spline S111 degree 2 poles (1.3284, -10.8984) (1.2466, -10.8408) (1.001, -10.8408) knots 0 0 0 1 1 1
  spline S112 degree 2 poles (1.001, -10.8408) (0.7541, -10.8408) (0.6729, -10.8984) knots 0 0 0 1 1 1
  spline S113 degree 2 poles (0.6729, -10.8984) (0.5917, -10.9561) (0.5917, -11.042) knots 0 0 0 1 1 1
  spline S114 degree 2 poles (0.5917, -11.042) (0.5917, -11.1266) (0.6634, -11.1771) knots 0 0 0 1 1 1
  spline S115 degree 2 poles (0.6634, -11.1771) (0.7548, -11.2405) (1.001, -11.2405) knots 0 0 0 1 1 1
  spline S116 degree 2 poles (1.001, -10.5898) (0.8237, -10.5898) (0.7156, -10.5533) knots 0 0 0 1 1 1
  spline S117 degree 2 poles (0.7156, -10.5533) (0.6074, -10.5168) (0.5488, -10.4448) knots 0 0 0 1 1 1
  spline S118 degree 2 poles (0.5488, -10.4448) (0.4901, -10.3728) (0.4901, -10.2637) knots 0 0 0 1 1 1
  spline S119 degree 2 poles (0.4901, -10.2637) (0.4901, -10.1832) (0.5225, -10.1225) knots 0 0 0 1 1 1
  spline S120 degree 2 poles (0.5225, -10.1225) (0.5549, -10.0618) (0.616, -10.0222) knots 0 0 0 1 1 1
  spline S121 degree 2 poles (0.616, -10.0222) (0.677, -9.9827) (0.7647, -9.9602) knots 0 0 0 1 1 1
  spline S122 degree 2 poles (0.7647, -9.9602) (0.8523, -9.9376) (1.001, -9.9376) knots 0 0 0 1 1 1
  spline S123 degree 2 poles (1.001, -9.9376) (1.177, -9.9376) (1.2851, -9.9738) knots 0 0 0 1 1 1
  spline S124 degree 2 poles (1.2851, -9.9738) (1.3933, -10.01) (1.4523, -10.0819) knots 0 0 0 1 1 1
  spline S125 degree 2 poles (1.4523, -10.0819) (1.5113, -10.1539) (1.5113, -10.2637) knots 0 0 0 1 1 1
  spline S126 degree 2 poles (1.5113, -10.2637) (1.5113, -10.4083) (1.4076, -10.4909) knots 0 0 0 1 1 1
  spline S127 degree 2 poles (1.4076, -10.4909) (1.2827, -10.5898) (1.001, -10.5898) knots 0 0 0 1 1 1
  spline S128 degree 2 poles (1.001, -10.4636) (1.2473, -10.4636) (1.3288, -10.4059) knots 0 0 0 1 1 1
  spline S129 degree 2 poles (1.3288, -10.4059) (1.4103, -10.3483) (1.4103, -10.2637) knots 0 0 0 1 1 1
  spline S130 degree 2 poles (1.4103, -10.2637) (1.4103, -10.1791) (1.3284, -10.1215) knots 0 0 0 1 1 1
  spline S131 degree 2 poles (1.3284, -10.1215) (1.2466, -10.0638) (1.001, -10.0638) knots 0 0 0 1 1 1
  spline S132 degree 2 poles (1.001, -10.0638) (0.7541, -10.0638) (0.6729, -10.1215) knots 0 0 0 1 1 1
  spline S133 degree 2 poles (0.6729, -10.1215) (0.5917, -10.1791) (0.5917, -10.2651) knots 0 0 0 1 1 1
  spline S134 degree 2 poles (0.5917, -10.2651) (0.5917, -10.3497) (0.6634, -10.4001) knots 0 0 0 1 1 1
  spline S135 degree 2 poles (0.6634, -10.4001) (0.7548, -10.4636) (1.001, -10.4636) knots 0 0 0 1 1 1
  line L45 (1.4942, -9.304) -> (1.3878, -9.304)
  spline S136 degree 2 poles (1.3878, -9.304) (1.5106, -9.3885) (1.5106, -9.5338) knots 0 0 0 1 1 1
  spline S137 degree 2 poles (1.5106, -9.5338) (1.5106, -9.5979) (1.486, -9.6535) knots 0 0 0 1 1 1
  spline S138 degree 2 poles (1.486, -9.6535) (1.4615, -9.7091) (1.4243, -9.7361) knots 0 0 0 1 1 1
  spline S139 degree 2 poles (1.4243, -9.7361) (1.3871, -9.763) (1.3332, -9.7739) knots 0 0 0 1 1 1
  spline S140 degree 2 poles (1.3332, -9.7739) (1.2971, -9.7814) (1.2186, -9.7814) knots 0 0 0 1 1 1
  line L46 (1.2186, -9.7814) -> (0.7698, -9.7814)
  line L47 (0.7698, -9.7814) -> (0.7698, -9.6587)
  line L48 (0.7698, -9.6587) -> (1.1716, -9.6587)
  spline S141 degree 2 poles (1.1716, -9.6587) (1.2677, -9.6587) (1.3012, -9.6512) knots 0 0 0 1 1 1
  spline S142 degree 2 poles (1.3012, -9.6512) (1.3496, -9.6396) (1.3772, -9.602) knots 0 0 0 1 1 1
  spline S143 degree 2 poles (1.3772, -9.602) (1.4048, -9.5645) (1.4048, -9.5093) knots 0 0 0 1 1 1
  spline S144 degree 2 poles (1.4048, -9.5093) (1.4048, -9.454) (1.3765, -9.4056) knots 0 0 0 1 1 1
  spline S145 degree 2 poles (1.3765, -9.4056) (1.3482, -9.3572) (1.2995, -9.337) knots 0 0 0 1 1 1
  spline S146 degree 2 poles (1.2995, -9.337) (1.2507, -9.3169) (1.1579, -9.3169) knots 0 0 0 1 1 1
  line L49 (1.1579, -9.3169) -> (0.7698, -9.3169)
  line L50 (0.7698, -9.3169) -> (0.7698, -9.1941)
  line L51 (0.7698, -9.1941) -> (1.4942, -9.1941)
  line L52 (1.4942, -9.1941) -> (1.4942, -9.304)
  line L53 (1.4942, -9.0018) -> (0.7698, -9.0018)
  line L54 (0.7698, -9.0018) -> (0.7698, -8.8919)
  line L55 (0.7698, -8.8919) -> (0.8714, -8.8919)
  spline S147 degree 2 poles (0.8714, -8.8919) (0.8182, -8.8578) (0.7858, -8.8012) knots 0 0 0 1 1 1
  spline S148 degree 2 poles (0.7858, -8.8012) (0.7534, -8.7446) (0.7534, -8.6723) knots 0 0 0 1 1 1
  spline S149 degree 2 poles (0.7534, -8.6723) (0.7534, -8.5918) (0.7868, -8.5403) knots 0 0 0 1 1 1
  spline S150 degree 2 poles (0.7868, -8.5403) (0.8203, -8.4888) (0.8803, -8.4677) knots 0 0 0 1 1 1
  spline S151 degree 2 poles (0.8803, -8.4677) (0.7534, -8.3817) (0.7534, -8.2439) knots 0 0 0 1 1 1
  spline S152 degree 2 poles (0.7534, -8.2439) (0.7534, -8.1361) (0.8131, -8.0782) knots 0 0 0 1 1 1
  spline S153 degree 2 poles (0.8131, -8.0782) (0.8728, -8.0202) (0.9969, -8.0202) knots 0 0 0 1 1 1
  line L56 (0.9969, -8.0202) -> (1.4942, -8.0202)
  line L57 (1.4942, -8.0202) -> (1.4942, -8.1423)
  line L58 (1.4942, -8.1423) -> (1.0379, -8.1423)
  spline S154 degree 2 poles (1.0379, -8.1423) (0.9642, -8.1423) (0.9318, -8.1542) knots 0 0 0 1 1 1
  spline S155 degree 2 poles (0.9318, -8.1542) (0.8994, -8.1662) (0.8796, -8.1975) knots 0 0 0 1 1 1
  spline S156 degree 2 poles (0.8796, -8.1975) (0.8598, -8.2289) (0.8598, -8.2712) knots 0 0 0 1 1 1
  spline S157 degree 2 poles (0.8598, -8.2712) (0.8598, -8.3476) (0.9106, -8.3981) knots 0 0 0 1 1 1
  spline S158 degree 2 poles (0.9106, -8.3981) (0.9615, -8.4486) (1.0733, -8.4486) knots 0 0 0 1 1 1
  line L59 (1.0733, -8.4486) -> (1.4942, -8.4486)
  line L60 (1.4942, -8.4486) -> (1.4942, -8.5713)
  line L61 (1.4942, -8.5713) -> (1.0235, -8.5713)
  spline S159 degree 2 poles (1.0235, -8.5713) (0.9417, -8.5713) (0.9008, -8.6014) knots 0 0 0 1 1 1
  spline S160 degree 2 poles (0.9008, -8.6014) (0.8598, -8.6314) (0.8598, -8.6996) knots 0 0 0 1 1 1
  spline S161 degree 2 poles (0.8598, -8.6996) (0.8598, -8.7514) (0.8871, -8.7954) knots 0 0 0 1 1 1
  spline S162 degree 2 poles (0.8871, -8.7954) (0.9144, -8.8394) (0.9669, -8.8592) knots 0 0 0 1 1 1
  spline S163 degree 2 poles (0.9669, -8.8592) (1.0194, -8.879) (1.1184, -8.879) knots 0 0 0 1 1 1
  line L62 (1.1184, -8.879) -> (1.4942, -8.879)
  line L63 (1.4942, -8.879) -> (1.4942, -9.0018)
  line L64 (1.4942, -7.514) -> (1.3714, -7.514)
  line L65 (1.3714, -7.514) -> (0.7309, -7.0018)
  spline S164 degree 2 poles (0.7309, -7.0018) (0.6627, -6.9472) (0.6122, -6.8981) knots 0 0 0 1 1 1
  line L66 (0.6122, -6.8981) -> (0.6122, -7.4561)
  line L67 (0.6122, -7.4561) -> (0.4942, -7.4561)
  line L68 (0.4942, -7.4561) -> (0.4942, -6.7398)
  line L69 (0.4942, -6.7398) -> (0.6122, -6.7398)
  line L70 (0.6122, -6.7398) -> (1.3059, -7.3012)
  line L71 (1.3059, -7.3012) -> (1.3762, -7.3619)
  line L72 (1.3762, -7.3619) -> (1.3762, -6.7235)
  line L73 (1.3762, -6.7235) -> (1.4942, -6.7235)
  line L74 (1.4942, -6.7235) -> (1.4942, -7.514)
  line L75 (23.4942, -5.3567) -> (23.4942, -5.2339)
  line L76 (23.4942, -5.2339) -> (24.2766, -5.2339)
  spline S165 degree 2 poles (24.2766, -5.2339) (24.2343, -5.1895) (24.192, -5.1176) knots 0 0 0 1 1 1
  spline S166 degree 2 poles (24.192, -5.1176) (24.1497, -5.0456) (24.1286, -4.9883) knots 0 0 0 1 1 1
  line L77 (24.1286, -4.9883) -> (24.2473, -4.9883)
  spline S167 degree 2 poles (24.2473, -4.9883) (24.2957, -5.0913) (24.3646, -5.1684) knots 0 0 0 1 1 1
  spline S168 degree 2 poles (24.3646, -5.1684) (24.4335, -5.2455) (24.4983, -5.2775) knots 0 0 0 1 1 1
  line L78 (24.4983, -5.2775) -> (24.4983, -5.3567)
  line L79 (24.4983, -5.3567) -> (23.4942, -5.3567)
  spline S169 degree 2 poles (23.9874, -5.6711) (24.1647, -5.6711) (24.2729, -5.7076) knots 0 0 0 1 1 1
  spline S170 degree 2 poles (24.2729, -5.7076) (24.381, -5.7441) (24.4396, -5.8161) knots 0 0 0 1 1 1
  spline S171 degree 2 poles (24.4396, -5.8161) (24.4983, -5.888) (24.4983, -5.9972) knots 0 0 0 1 1 1
  spline S172 degree 2 poles (24.4983, -5.9972) (24.4983, -6.0777) (24.4659, -6.1384) knots 0 0 0 1 1 1
  spline S173 degree 2 poles (24.4659, -6.1384) (24.4335, -6.1991) (24.3724, -6.2387) knots 0 0 0 1 1 1
  spline S174 degree 2 poles (24.3724, -6.2387) (24.3114, -6.2782) (24.2237, -6.3007) knots 0 0 0 1 1 1
  spline S175 degree 2 poles (24.2237, -6.3007) (24.1361, -6.3232) (23.9874, -6.3232) knots 0 0 0 1 1 1
  spline S176 degree 2 poles (23.9874, -6.3232) (23.8114, -6.3232) (23.7033, -6.2871) knots 0 0 0 1 1 1
  spline S177 degree 2 poles (23.7033, -6.2871) (23.5952, -6.2509) (23.5362, -6.179) knots 0 0 0 1 1 1
  spline S178 degree 2 poles (23.5362, -6.179) (23.4772, -6.107) (23.4772, -5.9972) knots 0 0 0 1 1 1
  spline S179 degree 2 poles (23.4772, -5.9972) (23.4772, -5.8526) (23.5808, -5.77) knots 0 0 0 1 1 1
  spline S180 degree 2 poles (23.5808, -5.77) (23.7057, -5.6711) (23.9874, -5.6711) knots 0 0 0 1 1 1
  spline S181 degree 2 poles (23.9874, -5.7973) (23.7411, -5.7973) (23.6596, -5.855) knots 0 0 0 1 1 1
  spline S182 degree 2 poles (23.6596, -5.855) (23.5781, -5.9126) (23.5781, -5.9972) knots 0 0 0 1 1 1
  spline S183 degree 2 poles (23.5781, -5.9972) (23.5781, -6.0818) (23.66, -6.1394) knots 0 0 0 1 1 1
  spline S184 degree 2 poles (23.66, -6.1394) (23.7418, -6.197) (23.9874, -6.197) knots 0 0 0 1 1 1
  spline S185 degree 2 poles (23.9874, -6.197) (24.2343, -6.197) (24.3155, -6.1394) knots 0 0 0 1 1 1
  spline S186 degree 2 poles (24.3155, -6.1394) (24.3967, -6.0818) (24.3967, -5.9958) knots 0 0 0 1 1 1
  spline S187 degree 2 poles (24.3967, -5.9958) (24.3967, -5.9112) (24.325, -5.8608) knots 0 0 0 1 1 1
  spline S188 degree 2 poles (24.325, -5.8608) (24.2336, -5.7973) (23.9874, -5.7973) knots 0 0 0 1 1 1
  spline S189 degree 2 poles (23.9874, -6.4481) (24.1647, -6.4481) (24.2729, -6.4846) knots 0 0 0 1 1 1
  spline S190 degree 2 poles (24.2729, -6.4846) (24.381, -6.5211) (24.4396, -6.593) knots 0 0 0 1 1 1
  spline S191 degree 2 poles (24.4396, -6.593) (24.4983, -6.665) (24.4983, -6.7741) knots 0 0 0 1 1 1
  spline S192 degree 2 poles (24.4983, -6.7741) (24.4983, -6.8546) (24.4659, -6.9153) knots 0 0 0 1 1 1
  spline S193 degree 2 poles (24.4659, -6.9153) (24.4335, -6.976) (24.3724, -7.0156) knots 0 0 0 1 1 1
  spline S194 degree 2 poles (24.3724, -7.0156) (24.3114, -7.0552) (24.2237, -7.0777) knots 0 0 0 1 1 1
  spline S195 degree 2 poles (24.2237, -7.0777) (24.1361, -7.1002) (23.9874, -7.1002) knots 0 0 0 1 1 1
  spline S196 degree 2 poles (23.9874, -7.1002) (23.8114, -7.1002) (23.7033, -7.064) knots 0 0 0 1 1 1
  spline S197 degree 2 poles (23.7033, -7.064) (23.5952, -7.0279) (23.5362, -6.9559) knots 0 0 0 1 1 1
  spline S198 degree 2 poles (23.5362, -6.9559) (23.4772, -6.8839) (23.4772, -6.7741) knots 0 0 0 1 1 1
  spline S199 degree 2 poles (23.4772, -6.7741) (23.4772, -6.6295) (23.5808, -6.547) knots 0 0 0 1 1 1
  spline S200 degree 2 poles (23.5808, -6.547) (23.7057, -6.4481) (23.9874, -6.4481) knots 0 0 0 1 1 1
  spline S201 degree 2 poles (23.9874, -6.5743) (23.7411, -6.5743) (23.6596, -6.6319) knots 0 0 0 1 1 1
  spline S202 degree 2 poles (23.6596, -6.6319) (23.5781, -6.6895) (23.5781, -6.7741) knots 0 0 0 1 1 1
  spline S203 degree 2 poles (23.5781, -6.7741) (23.5781, -6.8587) (23.66, -6.9163) knots 0 0 0 1 1 1
  spline S204 degree 2 poles (23.66, -6.9163) (23.7418, -6.974) (23.9874, -6.974) knots 0 0 0 1 1 1
  spline S205 degree 2 poles (23.9874, -6.974) (24.2343, -6.974) (24.3155, -6.9163) knots 0 0 0 1 1 1
  spline S206 degree 2 poles (24.3155, -6.9163) (24.3967, -6.8587) (24.3967, -6.7728) knots 0 0 0 1 1 1
  spline S207 degree 2 poles (24.3967, -6.7728) (24.3967, -6.6882) (24.325, -6.6377) knots 0 0 0 1 1 1
  spline S208 degree 2 poles (24.325, -6.6377) (24.2336, -6.5743) (23.9874, -6.5743) knots 0 0 0 1 1 1
  line L80 (23.6122, -8.6466) -> (23.4942, -8.6466)
  line L81 (23.4942, -8.6466) -> (23.4942, -7.9856)
  spline S209 degree 2 poles (23.4942, -7.9856) (23.5385, -7.9842) (23.5795, -7.9999) knots 0 0 0 1 1 1
  spline S210 degree 2 poles (23.5795, -7.9999) (23.647, -8.0251) (23.7125, -8.0807) knots 0 0 0 1 1 1
  spline S211 degree 2 poles (23.7125, -8.0807) (23.778, -8.1363) (23.8639, -8.2414) knots 0 0 0 1 1 1
  spline S212 degree 2 poles (23.8639, -8.2414) (23.9976, -8.4044) (24.0757, -8.4617) knots 0 0 0 1 1 1
  spline S213 degree 2 poles (24.0757, -8.4617) (24.1538, -8.519) (24.2234, -8.519) knots 0 0 0 1 1 1
  spline S214 degree 2 poles (24.2234, -8.519) (24.2964, -8.519) (24.3465, -8.4668) knots 0 0 0 1 1 1
  spline S215 degree 2 poles (24.3465, -8.4668) (24.3967, -8.4146) (24.3967, -8.3307) knots 0 0 0 1 1 1
  spline S216 degree 2 poles (24.3967, -8.3307) (24.3967, -8.2421) (24.3435, -8.1889) knots 0 0 0 1 1 1
  spline S217 degree 2 poles (24.3435, -8.1889) (24.2902, -8.1357) (24.1961, -8.135) knots 0 0 0 1 1 1
  line L82 (24.1961, -8.135) -> (24.2091, -8.0088)
  spline S218 degree 2 poles (24.2091, -8.0088) (24.3503, -8.0217) (24.4243, -8.1063) knots 0 0 0 1 1 1
  spline S219 degree 2 poles (24.4243, -8.1063) (24.4983, -8.1909) (24.4983, -8.3335) knots 0 0 0 1 1 1
  spline S220 degree 2 poles (24.4983, -8.3335) (24.4983, -8.4774) (24.4185, -8.5613) knots 0 0 0 1 1 1
  spline S221 degree 2 poles (24.4185, -8.5613) (24.3387, -8.6452) (24.2207, -8.6452) knots 0 0 0 1 1 1
  spline S222 degree 2 poles (24.2207, -8.6452) (24.1606, -8.6452) (24.1027, -8.6206) knots 0 0 0 1 1 1
  spline S223 degree 2 poles (24.1027, -8.6206) (24.0447, -8.5961) (23.9806, -8.5391) knots 0 0 0 1 1 1
  spline S224 degree 2 poles (23.9806, -8.5391) (23.9164, -8.4822) (23.8046, -8.3498) knots 0 0 0 1 1 1
  spline S225 degree 2 poles (23.8046, -8.3498) (23.7118, -8.2393) (23.6787, -8.208) knots 0 0 0 1 1 1
  spline S226 degree 2 poles (23.6787, -8.208) (23.6456, -8.1766) (23.6122, -8.1561) knots 0 0 0 1 1 1
  line L83 (23.6122, -8.1561) -> (23.6122, -8.6466)
  spline S227 degree 2 poles (23.9874, -8.7782) (24.1647, -8.7782) (24.2729, -8.8147) knots 0 0 0 1 1 1
  spline S228 degree 2 poles (24.2729, -8.8147) (24.381, -8.8512) (24.4396, -8.9232) knots 0 0 0 1 1 1
  spline S229 degree 2 poles (24.4396, -8.9232) (24.4983, -8.9951) (24.4983, -9.1043) knots 0 0 0 1 1 1
  spline S230 degree 2 poles (24.4983, -9.1043) (24.4983, -9.1848) (24.4659, -9.2455) knots 0 0 0 1 1 1
  spline S231 degree 2 poles (24.4659, -9.2455) (24.4335, -9.3062) (24.3724, -9.3457) knots 0 0 0 1 1 1
  spline S232 degree 2 poles (24.3724, -9.3457) (24.3114, -9.3853) (24.2237, -9.4078) knots 0 0 0 1 1 1
  spline S233 degree 2 poles (24.2237, -9.4078) (24.1361, -9.4303) (23.9874, -9.4303) knots 0 0 0 1 1 1
  spline S234 degree 2 poles (23.9874, -9.4303) (23.8114, -9.4303) (23.7033, -9.3942) knots 0 0 0 1 1 1
  spline S235 degree 2 poles (23.7033, -9.3942) (23.5952, -9.358) (23.5362, -9.2861) knots 0 0 0 1 1 1
  spline S236 degree 2 poles (23.5362, -9.2861) (23.4772, -9.2141) (23.4772, -9.1043) knots 0 0 0 1 1 1
  spline S237 degree 2 poles (23.4772, -9.1043) (23.4772, -8.9597) (23.5808, -8.8771) knots 0 0 0 1 1 1
  spline S238 degree 2 poles (23.5808, -8.8771) (23.7057, -8.7782) (23.9874, -8.7782) knots 0 0 0 1 1 1
  spline S239 degree 2 poles (23.9874, -8.9044) (23.7411, -8.9044) (23.6596, -8.9621) knots 0 0 0 1 1 1
  spline S240 degree 2 poles (23.6596, -8.9621) (23.5781, -9.0197) (23.5781, -9.1043) knots 0 0 0 1 1 1
  spline S241 degree 2 poles (23.5781, -9.1043) (23.5781, -9.1889) (23.66, -9.2465) knots 0 0 0 1 1 1
  spline S242 degree 2 poles (23.66, -9.2465) (23.7418, -9.3041) (23.9874, -9.3041) knots 0 0 0 1 1 1
  spline S243 degree 2 poles (23.9874, -9.3041) (24.2343, -9.3041) (24.3155, -9.2465) knots 0 0 0 1 1 1
  spline S244 degree 2 poles (24.3155, -9.2465) (24.3967, -9.1889) (24.3967, -9.1029) knots 0 0 0 1 1 1
  spline S245 degree 2 poles (24.3967, -9.1029) (24.3967, -9.0183) (24.325, -8.9678) knots 0 0 0 1 1 1
  spline S246 degree 2 poles (24.325, -8.9678) (24.2336, -8.9044) (23.9874, -8.9044) knots 0 0 0 1 1 1
  spline S247 degree 2 poles (23.9874, -9.5552) (24.1647, -9.5552) (24.2729, -9.5917) knots 0 0 0 1 1 1
  spline S248 degree 2 poles (24.2729, -9.5917) (24.381, -9.6281) (24.4396, -9.7001) knots 0 0 0 1 1 1
  spline S249 degree 2 poles (24.4396, -9.7001) (24.4983, -9.7721) (24.4983, -9.8812) knots 0 0 0 1 1 1
  spline S250 degree 2 poles (24.4983, -9.8812) (24.4983, -9.9617) (24.4659, -10.0224) knots 0 0 0 1 1 1
  spline S251 degree 2 poles (24.4659, -10.0224) (24.4335, -10.0831) (24.3724, -10.1227) knots 0 0 0 1 1 1
  spline S252 degree 2 poles (24.3724, -10.1227) (24.3114, -10.1623) (24.2237, -10.1848) knots 0 0 0 1 1 1
  spline S253 degree 2 poles (24.2237, -10.1848) (24.1361, -10.2073) (23.9874, -10.2073) knots 0 0 0 1 1 1
  spline S254 degree 2 poles (23.9874, -10.2073) (23.8114, -10.2073) (23.7033, -10.1711) knots 0 0 0 1 1 1
  spline S255 degree 2 poles (23.7033, -10.1711) (23.5952, -10.135) (23.5362, -10.063) knots 0 0 0 1 1 1